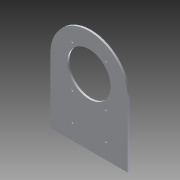
# Autodesk Inventor part: Top_Deck
Saved by Autodesk Inventor 2011 SP1 (Build 150282100, 282)
## iProperties
Created: 2011-06-12
Part Number: Top_Deck
Document SubType Name: Modeling
Designer: Andrew G. Meyer
Mass: 1353.83 g
Surface Area: 3074.37 cm^2
Volume: 1353.83 cm^3
Density: 1 g/cm^3
Author: Andrew G. Meyer
Autodesk Inventor part; units mm, degrees
ref_plane "YZ Plane" through (0, 0, 0) normal (1, 0, 0) x (0, 1, 0)
ref_plane "XZ Plane" through (0, 0, 0) normal (0, 1, 0) x (-1, 0, 0)
ref_plane "XY Plane" through (0, 0, 0) normal (0, 0, 1) x (1, 0, 0)
sketch "Sketch1" plane through (0, 0, 0) normal (0, 0, 1) x (1, 0, 0)
  line L0 (-190.5, -317.5) -> (190.5, -317.5)
  line L1 (190.5, -317.5) -> (190.5, 0)
  line L2 (-190.5, -317.5) -> (-190.5, 0)
  arc A0 (190.5, 0) -> (-190.5, 0) centre (0, 0) ccw
  dimension "d0" = 508
  dimension "d1" = 381
  constraints: 6 end point, 2 point on circle, 2 tangent, 1 centre point, 1 coincident, 1 horizontal, 1 parallel, 1 perpendicular
  measures "d1" distance of L0.start L0.end
extrude "Extrusion1" add sketch "Sketch1" along normal blind 9.525
hole "Hole1" at (82.55, -241.3, 9.525) direction (0, 0, -1) diameter 7.9375 depth 25.4 tip angle 118
hole "Hole2" at (-82.55, -241.3, 9.525) direction (0, 0, -1) diameter 7.9375 depth 25.4 tip angle 118
hole "Hole3" at (82.55, -104.775, 9.525) direction (0, 0, -1) diameter 7.9375 depth 25.4 tip angle 118
hole "Hole4" at (-82.55, -104.775, 9.525) direction (0, 0, -1) diameter 7.9375 depth 25.4 tip angle 118
hole "Hole5" at (-82.55, 101.6, 9.525) direction (0, 0, -1) diameter 7.9375 depth 25.4 tip angle 118
hole "Hole6" at (82.55, 101.6, 9.525) direction (0, 0, -1) diameter 7.9375 depth 25.4 tip angle 118
hole "Hole7" at (0, 6.35, 9.525) direction (0, 0, -1) diameter 212.725 depth 25.4 tip angle 118
body "Solid1"
